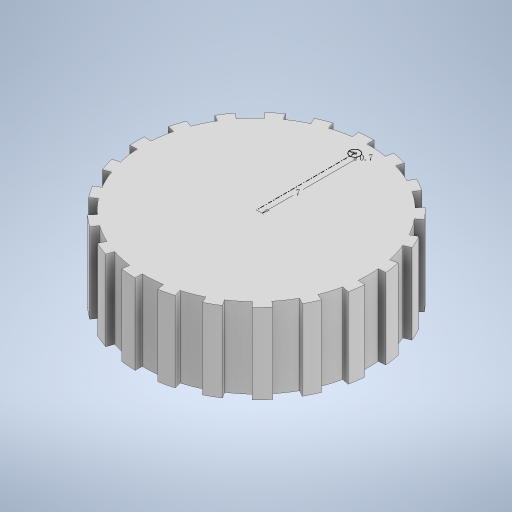
# Autodesk Inventor part: rot_no_val_sec_th
Saved by Autodesk Inventor 2023 (Build 270158000, 158)
## iProperties
Created: 2023-05-20
Part Number: rot_no_val_sec_th
Material: 常规
Document SubType Name: Modeling
Designer: LiuZeshu
Density: 1 g/cm^3
Appearance: 默认
Author: LiuZeshu
Autodesk Inventor part; units mm, degrees
ref_plane "YZ Plane" through (0, 0, 0) normal (1, 0, 0) x (0, 1, 0)
ref_plane "XZ Plane" through (0, 0, 0) normal (0, 1, 0) x (-1, 0, 0)
ref_plane "XY Plane" through (0, 0, 0) normal (0, 0, 1) x (1, 0, 0)
sketch "草图1" plane through (0, 0, 0) normal (0, 1, 0) x (-1, 0, 0)
  arc A0 (1.5875, -0.45) -> (-1.5875, -0.45) centre (0, 0) ccw
  line L0 (1.5875, -0.45) -> (-1.5875, -0.45)
  circle A1 centre (0, 0) radius 8
  dimension "d0" = 3.3
  dimension "d1" = 2.1
  dimension "d2" = 16
  constraints: 2 centre point, 2 coincident, 2 end point, 2 point on circle, 1 horizontal
  measures "d0" diameter of A0
  measures "d2" diameter of A1
extrude "拉伸1" add sketch "草图1" along normal blind 2.3
sketch "草图2" plane through (0, 2.3, 0) normal (0, 1, 0) x (1, 0, 0)
  circle A0 centre (0, 0) radius 8
  line L0 (-1.5875, 0.45) -> (1.5875, 0.45) projected
  arc A1 (-1.5875, 0.45) -> (1.5875, 0.45) centre (0, 0) ccw
  line L1 (-1.5875, 0.45) -> (1.5875, 0.45)
  circle A2 centre (0, 0) radius 8 projected
  constraints: 2 centre point, 2 coincident, 2 end point, 2 point on circle, 1 collinear, 1 concentric
extrude "拉伸2" add sketch "草图2" along normal blind 0.4 contours A0 | L0 A1
sketch "草图5" plane through (0, 2.7, 0) normal (0, 1, 0) x (1, 0, 0)
  circle A0 centre (0, 7) radius 0.35
  line L0 (0, 7) -> (0, 0)
  dimension "d27" = 0.7
  dimension "d28" = 7
  constraints: 2 end point, 1 centre point, 1 vertical
  measures "d27" diameter of A0
  measures "d28" distance of L0.end L0.start
sketch "草图7" plane through (0, 0, 0) normal (0, -1, 0) x (1, 0, 0)
  circle A0 centre (0, 0) radius 8
  circle A1 centre (0, 0) radius 8 projected
  circle A2 centre (0, 0) radius 6.35
  dimension "d39" = 12.7
  constraints: 2 centre point, 2 coincident, 1 concentric
  measures "d39" diameter of A2
extrude "拉伸7" add sketch "草图7" along normal blind 3
sketch "草图6" plane through (0, 2.7, 0) normal (0, 1, 0) x (1, 0, 0)
  arc A0 (-7.9851, 0.4884) -> (-7.9851, -0.4884) centre (0, 0) ccw
  circle A1 centre (0, 0) radius 8 projected
  arc A2 (-1.5875, 0.45) -> (1.5875, 0.45) centre (0, 0) ccw projected
  arc A3 (-8.4841, 0.5189) -> (-8.4841, -0.5189) centre (0, 0) ccw
  line L0 (-8.4841, -0.5189) -> (-7.9851, -0.4884)
  line L1 (-8.4841, 0.5189) -> (-7.9851, 0.4884)
  line L2 (-11.1138, 0) -> (0, 0)
  line L3 (-1.5875, 0.45) -> (1.5875, 0.45) projected
  arc A4 (-7.7743, -1.887) -> (-7.4864, -2.8203) centre (0, 0) ccw
  arc A5 (-8.2602, -2.0049) -> (-7.9543, -2.9966) centre (0, 0) ccw
  line L4 (-7.9543, -2.9966) -> (-7.4864, -2.8203)
  line L5 (-8.2602, -2.0049) -> (-7.7743, -1.887)
  line L6 (-10.62, -3.2758) -> (0, 0)
  arc A6 (-6.8727, -4.0946) -> (-6.3225, -4.9017) centre (0, 0) ccw
  arc A7 (-7.3022, -4.3505) -> (-6.7176, -5.208) centre (0, 0) ccw
  line L7 (-6.7176, -5.208) -> (-6.3225, -4.9017)
  line L8 (-7.3022, -4.3505) -> (-6.8727, -4.0946)
  line L9 (-9.1826, -6.2606) -> (0, 0)
  arc A8 (-5.3605, -5.9385) -> (-4.5968, -6.5475) centre (0, 0) ccw
  arc A9 (-5.6955, -6.3096) -> (-4.8841, -6.9567) centre (0, 0) ccw
  line L10 (-4.8841, -6.9567) -> (-4.5968, -6.5475)
  line L11 (-5.6955, -6.3096) -> (-5.3605, -5.9385)
  line L12 (-6.9293, -8.6891) -> (0, 0)
  arc A10 (-3.3719, -7.2547) -> (-2.4626, -7.6115) centre (0, 0) ccw
  arc A11 (-3.5826, -7.7081) -> (-2.6166, -8.0872) centre (0, 0) ccw
  line L13 (-2.6166, -8.0872) -> (-2.4626, -7.6115)
  line L14 (-3.5826, -7.7081) -> (-3.3719, -7.2547)
  line L15 (-4.0603, -10.3455) -> (0, 0)
  arc A12 (-1.0837, -7.9263) -> (-0.1097, -7.9992) centre (0, 0) ccw
  arc A13 (-1.1515, -8.4216) -> (-0.1166, -8.4992) centre (0, 0) ccw
  line L16 (-0.1166, -8.4992) -> (-0.1097, -7.9992)
  line L17 (-1.1515, -8.4216) -> (-1.0837, -7.9263)
  line L18 (-0.8305, -11.0827) -> (0, 0)
  arc A14 (1.3007, -7.8936) -> (2.253, -7.6762) centre (0, 0) ccw
  arc A15 (1.382, -8.3869) -> (2.3938, -8.156) centre (0, 0) ccw
  line L19 (2.3938, -8.156) -> (2.253, -7.6762)
  line L20 (1.382, -8.3869) -> (1.3007, -7.8936)
  line L21 (2.4731, -10.8351) -> (0, 0)
  arc A16 (3.5696, -7.1595) -> (4.4155, -6.6711) centre (0, 0) ccw
  arc A17 (3.7927, -7.6069) -> (4.6915, -7.088) centre (0, 0) ccw
  line L22 (4.6915, -7.088) -> (4.4155, -6.6711)
  line L23 (3.7927, -7.6069) -> (3.5696, -7.1595)
  line L24 (5.5569, -9.6248) -> (0, 0)
  arc A18 (5.5213, -5.7892) -> (6.1857, -5.0732) centre (0, 0) ccw
  arc A19 (5.8664, -6.1511) -> (6.5723, -5.3903) centre (0, 0) ccw
  line L25 (6.5723, -5.3903) -> (6.1857, -5.0732)
  line L26 (5.8664, -6.1511) -> (5.5213, -5.7892)
  line L27 (8.147, -7.5593) -> (0, 0)
  arc A20 (6.9824, -3.9046) -> (7.4062, -3.0246) centre (0, 0) ccw
  arc A21 (7.4188, -4.1487) -> (7.8691, -3.2136) centre (0, 0) ccw
  line L28 (7.8691, -3.2136) -> (7.4062, -3.0246)
  line L29 (7.4188, -4.1487) -> (6.9824, -3.9046)
  line L30 (10.0132, -4.8221) -> (0, 0)
  arc A22 (7.8231, -1.673) -> (7.9687, -0.7072) centre (0, 0) ccw
  arc A23 (8.312, -1.7776) -> (8.4667, -0.7514) centre (0, 0) ccw
  line L31 (8.4667, -0.7514) -> (7.9687, -0.7072)
  line L32 (8.312, -1.7776) -> (7.8231, -1.673)
  line L33 (10.9897, -1.6564) -> (0, 0)
  arc A24 (7.9687, 0.7072) -> (7.8231, 1.673) centre (0, 0) ccw
  arc A25 (8.4667, 0.7514) -> (8.312, 1.7776) centre (0, 0) ccw
  line L34 (8.312, 1.7776) -> (7.8231, 1.673)
  line L35 (8.4667, 0.7514) -> (7.9687, 0.7072)
  line L36 (10.9897, 1.6564) -> (0, 0)
  arc A26 (7.4062, 3.0246) -> (6.9824, 3.9046) centre (0, 0) ccw
  arc A27 (7.8691, 3.2136) -> (7.4188, 4.1487) centre (0, 0) ccw
  line L37 (7.4188, 4.1487) -> (6.9824, 3.9046)
  line L38 (7.8691, 3.2136) -> (7.4062, 3.0246)
  line L39 (10.0132, 4.8221) -> (0, 0)
  arc A28 (6.1857, 5.0732) -> (5.5213, 5.7892) centre (0, 0) ccw
  arc A29 (6.5723, 5.3903) -> (5.8664, 6.1511) centre (0, 0) ccw
  line L40 (5.8664, 6.1511) -> (5.5213, 5.7892)
  line L41 (6.5723, 5.3903) -> (6.1857, 5.0732)
  line L42 (8.147, 7.5593) -> (0, 0)
  arc A30 (4.4155, 6.6711) -> (3.5696, 7.1595) centre (0, 0) ccw
  arc A31 (4.6915, 7.088) -> (3.7927, 7.6069) centre (0, 0) ccw
  line L43 (3.7927, 7.6069) -> (3.5696, 7.1595)
  line L44 (4.6915, 7.088) -> (4.4155, 6.6711)
  line L45 (5.5569, 9.6248) -> (0, 0)
  arc A32 (2.253, 7.6762) -> (1.3007, 7.8936) centre (0, 0) ccw
  arc A33 (2.3938, 8.156) -> (1.382, 8.3869) centre (0, 0) ccw
  line L46 (1.382, 8.3869) -> (1.3007, 7.8936)
  line L47 (2.3938, 8.156) -> (2.253, 7.6762)
  line L48 (2.4731, 10.8351) -> (0, 0)
  arc A34 (-0.1097, 7.9992) -> (-1.0837, 7.9263) centre (0, 0) ccw
  arc A35 (-0.1166, 8.4992) -> (-1.1515, 8.4216) centre (0, 0) ccw
  line L49 (-1.1515, 8.4216) -> (-1.0837, 7.9263)
  line L50 (-0.1166, 8.4992) -> (-0.1097, 7.9992)
  line L51 (-0.8305, 11.0827) -> (0, 0)
  arc A36 (-2.4626, 7.6115) -> (-3.3719, 7.2547) centre (0, 0) ccw
  arc A37 (-2.6166, 8.0872) -> (-3.5826, 7.7081) centre (0, 0) ccw
  line L52 (-3.5826, 7.7081) -> (-3.3719, 7.2547)
  line L53 (-2.6166, 8.0872) -> (-2.4626, 7.6115)
  line L54 (-4.0603, 10.3455) -> (0, 0)
  arc A38 (-4.5968, 6.5475) -> (-5.3605, 5.9385) centre (0, 0) ccw
  arc A39 (-4.8841, 6.9567) -> (-5.6955, 6.3096) centre (0, 0) ccw
  line L55 (-5.6955, 6.3096) -> (-5.3605, 5.9385)
  line L56 (-4.8841, 6.9567) -> (-4.5968, 6.5475)
  line L57 (-6.9293, 8.6891) -> (0, 0)
  arc A40 (-6.3225, 4.9017) -> (-6.8727, 4.0946) centre (0, 0) ccw
  arc A41 (-6.7176, 5.208) -> (-7.3022, 4.3505) centre (0, 0) ccw
  line L58 (-7.3022, 4.3505) -> (-6.8727, 4.0946)
  line L59 (-6.7176, 5.208) -> (-6.3225, 4.9017)
  line L60 (-9.1826, 6.2606) -> (0, 0)
  arc A42 (-7.4864, 2.8203) -> (-7.7743, 1.887) centre (0, 0) ccw
  arc A43 (-7.9543, 2.9966) -> (-8.2602, 2.0049) centre (0, 0) ccw
  line L61 (-8.2602, 2.0049) -> (-7.7743, 1.887)
  line L62 (-7.9543, 2.9966) -> (-7.4864, 2.8203)
  line L63 (-10.62, 3.2758) -> (0, 0)
  point P0 (6.9824, 3.9046)
  point P1 (7.4062, 3.0246)
  point P2 (5.5213, 5.7892)
  point P3 (6.1857, 5.0732)
  point P4 (3.5696, 7.1595)
  point P5 (4.4155, 6.6711)
  point P6 (1.3007, 7.8936)
  point P7 (2.253, 7.6762)
  point P8 (-1.0837, 7.9263)
  point P9 (-3.3719, 7.2547)
  point P10 (-2.4626, 7.6115)
  point P11 (-5.3605, 5.9385)
  point P12 (-4.5968, 6.5475)
  point P13 (-6.8727, 4.0946)
  point P14 (-6.3225, 4.9017)
  point P15 (-7.4864, 2.8203)
  point P16 (-7.4864, -2.8203)
  point P17 (-7.7743, -1.887)
  point P18 (-6.3225, -4.9017)
  point P19 (-6.8727, -4.0946)
  point P20 (-4.5968, -6.5475)
  point P21 (-5.3605, -5.9385)
  point P22 (-2.4626, -7.6115)
  point P23 (-3.3719, -7.2547)
  point P24 (-0.1097, -7.9992)
  point P25 (-1.0837, -7.9263)
  point P26 (2.253, -7.6762)
  point P27 (1.3007, -7.8936)
  point P28 (4.4155, -6.6711)
  point P29 (3.5696, -7.1595)
  point P30 (6.1857, -5.0732)
  point P31 (5.5213, -5.7892)
  point P32 (7.4062, -3.0246)
  point P33 (6.9824, -3.9046)
  point P34 (7.9687, -0.7072)
  point P35 (7.8231, -1.673)
  point P36 (7.8231, 1.673)
  point P37 (7.9687, 0.7072)
  dimension "d31" = 0.5
  dimension "d32" = 7
  dimension "d35" = 360
  constraints: 126 end point, 84 point on circle, 44 coincident, 42 centre point, 42 point on line, 1 parallel, 298 other
  measures "d31" radial gap between concentric circles of A3 A0
  measures "d32" angle of L1 L0
extrude "拉伸6" add sketch "草图6" against normal up to surface (5.7 mm away) contours A0 L2 A3 L1 | A0 L0 A3 L2 | L61 A43 L63 A1 | L63 A43 L62 A1 | A1 L6 A5 L5 | A1 L4 A5 L6 | L58 A41 L60 A1 | L9 A7 L8 A1 | A1 L7 A7 L9 | L12 A9 L11 A1 | A1 L10 A9 L12 | L15 A11 L14 A1 | A1 L13 A11 L15 | L18 A13 L17 A1 | A1 L16 A13 L18 | L21 A15 L20 A1 | A1 L19 A15 L21 | L24 A17 L23 A1 | A1 L22 A17 L24 | L27 A19 L26 A1 | A1 L25 A19 L27 | L30 A21 L29 A1 | A1 L28 A21 L30 | L33 A23 L32 A1 | A1 L31 A23 L33 | L36 A25 L35 A1 | A1 L34 A25 L36 | L39 A27 L38 A1 | A1 L37 A27 L39 | L42 A29 L41 A1 | A1 L40 A29 L42 | L45 A31 L44 A1 | A1 L43 A31 L45 | L48 A33 L47 A1 | A1 L46 A33 L48 | L51 A35 L50 A1 | A1 L49 A35 L51 | L54 A37 L53 A1 | A1 L52 A37 L54 | L57 A39 L56 A1 | A1 L55 A39 L57 | L60 A41 L59 A1
